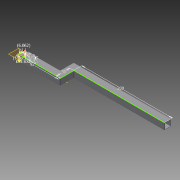
# Autodesk Inventor part: Alkar
Saved by Autodesk Inventor 2015 (Build 190159000, 159)
## iProperties
Created: 2014-09-09
Part Number: Alkar
Material: Generic
Document SubType Name: Modeling
Designer: laca
Density: 1 g/cm^3
Appearance: Default
Mass: 26.2776 g
Surface Area: 349.958 cm^2
Volume: 26.2776 cm^3
Author: laca
Autodesk Inventor part; units mm, degrees
ref_plane "YZ Plane" through (0, 0, 0) normal (1, 0, 0) x (0, 1, 0)
ref_plane "XZ Plane" through (0, 0, 0) normal (0, 1, 0) x (-1, 0, 0)
ref_plane "XY Plane" through (0, 0, 0) normal (0, 0, 1) x (1, 0, 0)
derived "KétvégenMartSzelvény.ipt"
sketch "Sketch1" plane through (0, 0, 0) normal (1, 0, 0) x (0, 1, 0)
  line L0 (0, 0) -> (12, 0)
  line L1 (12, 0) -> (12, 12)
  line L2 (12, 12) -> (0, 12)
  line L3 (0, 12) -> (0, 0)
  line L4 (-1.5, 13.5) -> (13.5, 13.5)
  line L5 (13.5, 13.5) -> (13.5, -1.5)
  line L6 (13.5, -1.5) -> (-1.5, -1.5)
  line L7 (-1.5, -1.5) -> (-1.5, 13.5)
  dimension "d33" = 15
  measures "d33" distance of L4.start L4.end
ref_plane "Work Plane1" through (0, 13.5, 13.5) normal (0, 1, 0) x (1, 0, 0)
sketch "Sketch3" plane through (0, 13.5, 13.5) normal (0, 1, 0) x (1, 0, 0)
  line L0 (0, 0) -> (92, 0)
  line L1 (92, 0) -> (92, 30)
  line L2 (92, 30) -> (292, 30)
  circle A0 centre (0, 7.5) radius 2
  point P0 (0, 13.5)
  dimension "d3" = 92
  dimension "d4" = 30
  dimension "d5" = 200
  dimension "d31" = 4
  dimension "d32" = 7.5
  constraints: 6 end point, 2 perpendicular, 1 centre point, 1 horizontal
  measures "d3" distance of L0.start L0.end
  measures "d4" distance of L0.end L1.end
  measures "d5" distance of L1.end L2.end
  measures "d31" diameter of A0
  measures "d32" distance from line of L0 A0.centre
sweep "Sweep1" add profiles "Sketch1" path "Sketch3" path curves L0 L1 L2
sketch "Sketch4" plane through (0, -1.5, -1.5) normal (0, 0, -1) x (-1, 0, 0)
  line L0 (0, 0) -> (-92, 0) projected
  line L1 (-6.0622, 0) -> (-6.0622, 15)
  line L2 (0, 14.5) -> (6.0622, 11)
  line L3 (6.0622, 11) -> (6.0622, 4)
  line L4 (6.0622, 4) -> (0, 0.5)
  line L5 (0, 0.5) -> (-6.0622, 4)
  line L6 (-6.0622, 4) -> (-6.0622, 11)
  line L7 (-6.0622, 11) -> (0, 14.5)
  line L8 (0, 15) -> (0, 0) projected
  circle A0 centre (0, 7.5) radius 5
  point P0 (0, 7.5)
  point P1 (-6.0622, 7.5)
  point P2 (-6.0622, 7.5)
  point P3 (-6.0622, 7.5)
  dimension "d9" = 7
  dimension "d10" = 3.5
  dimension "d11" = 7.5
  dimension "d12" = 15
  dimension "d13" = 6.0622
  dimension "d14" = 6.0622
  dimension "d15" = 10
  constraints: 14 end point, 4 midpoint, 1 centre point, 1 collinear, 1 point on line, 1 vertical, 13 other
  measures "d9" distance of L2.end L3.end
  measures "d10" distance of L6.end point (-6.062, 7.5)
  measures "d11" distance of L1.start point (-6.062, 7.5)
  measures "d12" distance of L1.start L1.end
  measures "d13" distance between parallel lines of L1 L8
  measures "d14" distance from line of L3 point (0, 7.5)
  measures "d15" diameter of A0
extrude "Extrusion2" cut sketch "Sketch4" against normal through all contours L8 A0 L2 L3 L4 | L5 L1 L7 L8 A0 | A0 L8 | L8 A0
extrude "Extrusion3" add sketch "Sketch4" against normal up to surface (15 mm away) contours L8 A0 L2 L3 L4 | L5 L1 L7 L8 A0
chamfer "Chamfer1" distance 0.5 angle 45 2 edges at (0, 13.5, 6) (0, -1.5, 6)
fillet "Fillet1" radius 2 4 edges at (92, 6, 13.5) (92, 6, -16.5) (77, 6, -1.5) (77, 6, -31.5)
fillet "Fillet2" radius 1 20 edges at (91.4142, 13.5, 12.9142) (92, 13.5, -1.5) (92.5858, 13.5, -15.9142) (193, 13.5, -16.5) (45.25, 13.5, 13.5) (76.4142, 13.5, -2.0858) (77, 13.5, -16.5) (77.5858, 13.5, -30.9142) (185.5, 13.5, -31.5) (37.75, 13.5, -1.5) (91.4142, -1.5, 12.9142) (92, -1.5, -1.5) (92.5858, -1.5, -15.9142) (193, -1.5, -16.5) (45.25, -1.5, 13.5) (76.4142, -1.5, -2.0858) (77, -1.5, -16.5) (77.5858, -1.5, -30.9142) (185.5, -1.5, -31.5) (37.75, -1.5, -1.5)
fillet "Fillet3" radius 1 8 edges at (292, 13.2071, -16.7929) (292, 6, -16.5) (292, -1.2071, -16.7929) (292, -1.5, -24) (292, -1.2071, -31.2071) (292, 6, -31.5) (292, 13.2071, -31.2071) (292, 13.5, -24)
thread "Thread1"
chamfer "Chamfer2" distance 1 angle 45 2 edges at (5, 6, -1.5) (5, 6, 13.5)
equation "\"d32\" = 0.5 * d33"
equation "\"d10\" = 0.5 * d9"
equation "\"d11\" = 0.5 * d12"
equation "\"d13\" = d14"
body "Solid2"
